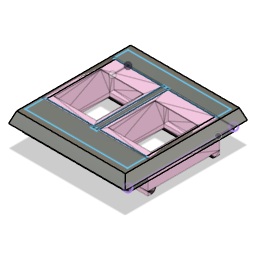
Pop Up Power Strip Keystone Adapter (Autodesk Fusion 360 design; units mm, degrees)
Autodesk Fusion 360 part; units mm, degrees
sketch "Sketch1" plane through (0, 0, 0) normal (0, 1, 0) x (1, 0, 0)
  line L0 (25, 25) -> (62, 25)
  line L1 (62, 25) -> (62, 62)
  line L2 (62, 62) -> (25, 62)
  line L3 (25, 62) -> (25, 25)
  line L4 (25, 25) -> (26.5, 25) construction
  line L5 (62, 62) -> (63.5, 62) construction
  line L6 (26.0607, 26.0607) -> (60.9393, 26.0607)
  line L7 (60.9393, 26.0607) -> (60.9393, 60.9393)
  line L8 (60.9393, 60.9393) -> (26.0607, 60.9393)
  line L9 (26.0607, 60.9393) -> (26.0607, 26.0607)
  line L10 (25, 62) -> (62, 25)
  line L11 (25, 25) -> (62, 62)
  point P0 (43.5, 43.5)
  dimension "d1" = 37
  dimension "d2" = 37
  dimension "d3" = 1.5
  dimension "d6" = 1.5
  constraint horizontal L0
  constraint vertical L1
  constraint horizontal L2
  constraint vertical L3
  constraint horizontal L4
  constraint horizontal L5
  constraint horizontal L6
  constraint vertical L7
  constraint horizontal L8
  constraint vertical L9
  constraint midpoint L10 P0
  measures "d1" distance of L0.start L0.end
  measures "d2" distance of L0.start L2.end
  measures "d3" distance of L0.start L6.start
  measures "d6" distance of L1.end L7.end
extrude "Extrude1" add sketch "Sketch1" along normal blind 1.5 contours L0 L6 L10 L11 | L3 L9 L10 L11 | L1 L7 L10 L11 | L2 L8 L10 L11 makes body 1
sketch "Sketch3" plane through (0, 0, 0) normal (0, 1, 0) x (1, 0, 0)
  line L0 (23.125, 22.125, 1.5) -> (63.875, 22.125, 1.5)
  line L1 (63.875, 22.125, 1.5) -> (63.875, 64.875, 1.5)
  line L2 (63.875, 64.875, 1.5) -> (23.125, 64.875, 1.5)
  line L3 (23.125, 64.875, 1.5) -> (23.125, 22.125, 1.5)
  point P0 (43.5, 43.5)
  point P1 (23.125, 22.125)
  point P2 (63.875, 22.125)
  point P3 (23.125, 64.875)
  point P4 (63.875, 64.875)
  dimension "d9" = 40.75
  dimension "d10" = 42.75
  measures "d9" distance of P1 P2
  measures "d10" distance of P1 P3
sketch "Sketch4" plane through (0, 0, 0) normal (0, 1, 0) x (1, 0, 0)
  line L0 (24.5049, 23.5727, 5.25) -> (62.4951, 23.5727, 5.25)
  line L1 (62.4951, 23.5727, 5.25) -> (62.4951, 63.4273, 5.25)
  line L2 (62.4951, 63.4273, 5.25) -> (24.5049, 63.4273, 5.25)
  line L3 (24.5049, 63.4273, 5.25) -> (24.5049, 23.5727, 5.25)
extrude "Extrude2" add 1 faces at (37.6869, 1.5, -25.3536) along direction (0, 1, 0) blind 3.75 on bodies 1 bodies 1
loft "Loft1" add profiles "Sketch4", "Sketch3" section 1 contours L0 L1 L2 L3 in plane through (0, 5.25, 0) normal (0, 1, 0) section 2 contours L0 L1 L2 L3 in plane through (0, 1.5, 0) normal (0, 1, 0) separate body makes body 2
sketch "Sketch5" plane through (0, 0, 0) normal (0, 1, 0) x (1, 0, 0)
  line L0 (26.0607, 60.9393) -> (60.9393, 60.9393)
  line L1 (60.9393, 60.9393) -> (60.9393, 26.0607)
  line L2 (60.9393, 26.0607) -> (26.0607, 26.0607)
  line L3 (26.0607, 26.0607) -> (26.0607, 60.9393)
  point P0 (26.0607, 60.9393)
  point P1 (60.9393, 26.0607)
  constraint horizontal L0
  constraint vertical L1
  constraint horizontal L2
  constraint vertical L3
  constraint coincident P1 L1.end
  constraint coincident P0 L0.start
extrude "Extrude3" cut sketch "Sketch5" along normal blind 15 bodies 2
extrude "Extrude4" add 1 faces at (37.6869, 0, -25.3536) along direction (0, -1, 0) blind 1.5 on bodies 1 bodies 1
other "Base Mesh Feature1"
other "Modify1"
other "Modify2"
other "CopyPasteMeshes1"
other "Modify3"
other "Modify4"
other "Modify5"
other "Modify6"
sketch "Sketch6" plane through (0, 0, 0) normal (0, 1, 0) x (1, 0, 0)
  line L0 (25, 62) -> (62, 62)
  line L1 (62, 62) -> (62, 56.5153)
  line L2 (25, 56.5153) -> (25, 62)
  line L3 (62, 25) -> (62, 62)
  line L4 (42.5, 57, 5.25) -> (44.5, 57, 5.25)
  line L5 (44.5, 57, 5.25) -> (44.5, 31.5, 5.25)
  line L6 (44.5, 31.5, 5.25) -> (42.5, 31.5, 5.25)
  line L7 (42.5, 31.5, 5.25) -> (42.5, 57, 5.25)
  line L8 (61.4138, 56.5153, 5.25) -> (25.5, 56.5153, 5.25)
  line L9 (25.5, 56.5153, 5.25) -> (25.5, 61.5, 5.25)
  line L10 (25.5, 61.5, 5.25) -> (61.4138, 61.5, 5.25)
  line L11 (61.4138, 61.5, 5.25) -> (61.4138, 56.5153, 5.25)
  line L12 (61.2339, 25.5838, 5.25) -> (25.4824, 25.5838, 5.25)
  line L13 (25.4824, 25.5838, 5.25) -> (25.4824, 32.4652, 5.25)
  line L14 (25.4824, 32.4652, 5.25) -> (61.2339, 32.4652, 5.25)
  line L15 (61.2339, 32.4652, 5.25) -> (61.2339, 25.5838, 5.25)
  point P0 (25, 62)
  constraint horizontal L0
  constraint vertical L1
  constraint vertical L2
  constraint coincident L1.end L3
  constraint coincident P0 L0.start
extrude "Extrude5" add sketch "Sketch6" against normal blind 1.5 contours L4 L5 L7 L8 L9 L10 L11 | L5 L7 L8 L14 | L5 L6 L7 L14 | L5 L6 L7 L12 L13 L14 L15 in plane through (0, 5.25, 0) normal (0, 1, 0) bodies 1 2
extrude "Extrude6" add sketch "Sketch6" against normal blind 1.5 contours L4 L5 L7 L8 in plane through (0, 5.25, 0) normal (0, 1, 0) bodies 1
